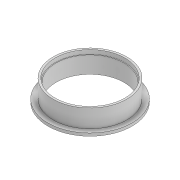
# Autodesk Inventor part: mask_breath_top_lc
Saved by Autodesk Inventor 2021 (Build 250183000, 183)
## iProperties
Created: 2020-04-13
Part Number: mask_breath_top_lc
Material: Generic
Document SubType Name: Modeling
Designer: Muchiri John
Density: 1 g/cm^3
Appearance: Default
Author: Muchiri John
Autodesk Inventor part; units mm, degrees
ref_plane "YZ Plane" through (0, 0, 0) normal (1, 0, 0) x (0, 1, 0)
ref_plane "XZ Plane" through (0, 0, 0) normal (0, 1, 0) x (-1, 0, 0)
ref_plane "XY Plane" through (0, 0, 0) normal (0, 0, 1) x (1, 0, 0)
sketch "Sketch1" plane through (0, 0, 0) normal (0, 0, 1) x (1, 0, 0)
  line L0 (10.8649, 4.9355) -> (14.8649, 4.9355)
  line L1 (13.4649, 6.3355) -> (10.8649, 6.3355)
  line L2 (10.8649, 6.3355) -> (10.8649, 4.9355)
  line L3 (13.4649, 6.3355) -> (13.4649, 15.3355)
  line L4 (13.4649, 15.3355) -> (14.4649, 15.3355)
  line L5 (14.4649, 15.3355) -> (14.4649, 13.3355)
  line L6 (14.4649, 13.3355) -> (14.8649, 13.3355)
  line L7 (14.8649, 13.3355) -> (14.8649, 4.9355)
  line L8 (31.8649, 18.7517) -> (31.8649, 1.3446)
  dimension "d4" = 9
  dimension "d6" = 1
  dimension "d7" = 2
  dimension "d10" = 0.4
  dimension "d12" = 8.4
  dimension "d13" = 21
  dimension "d15" = 18.4
  dimension "d17" = 1.4
  constraints: 18 end point, 2 horizontal, 2 perpendicular, 2 vertical, 1 parallel
  measures "d4" distance of L1.start L3.end
  measures "d6" distance of L3.end L4.end
  measures "d7" distance of L4.end L5.end
  measures "d10" distance of L5.end L6.end
  measures "d12" distance of L6.end L0.end
  measures "d13" distance between parallel lines of L8 L2
  measures "d15" distance between parallel lines of L3 L8
  measures "d17" distance of L1.end L0.start
revolve "Revolution1" add sketch "Sketch1" angle 360 about axis through (31.8649, 18.7517, 0) along (0, -1, 0)
body "Solid1"
